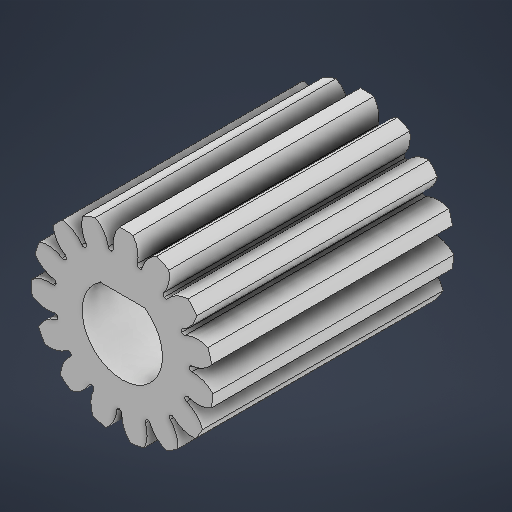
# Autodesk Inventor part: piñon
Saved by Autodesk Inventor 2025.3 (Build 293356000, 356)
## iProperties
Created: 2024-05-16
Part Number: piñon
Material: Genérico
Document SubType Name: Modeling
Designer: Jonathan Galarza
Density: 1 g/cm^3
Appearance: Valor por defecto
Author: Jonathan Galarza
Title: Eje piñon
Autodesk Inventor part; units mm, degrees
ref_plane "YZ Plane" through (0, 0, 0) normal (1, 0, 0) x (0, 1, 0)
ref_plane "XZ Plane" through (0, 0, 0) normal (0, 1, 0) x (-1, 0, 0)
ref_plane "XY Plane" through (0, 0, 0) normal (0, 0, 1) x (1, 0, 0)
sketch "Boceto1" plane through (0, 0, 0) normal (0, 0, 1) x (1, 0, 0)
  circle A0 centre (0, 0) radius 17
  dimension "d0" = 34
  constraints: 1 centre point, 1 coincident
  measures "d0" diameter of A0
extrude "Extrusión1" add sketch "Boceto1" along normal blind 1
sketch "Boceto2" plane through (0, 0, 0) normal (0, 0, -1) x (-1, 0, 0)
  point P0 (0, 0)
sketch "Boceto6" plane through (0, 0, 1) normal (0, 0, 1) x (1, 0, 0)
  arc A0 (6.6315, -1.5044) -> (6.7809, -0.5097) centre (0, 0) ccw
  circle A1 centre (0, 0) radius 5
  line L0 (0, 0) -> (6.8, 0) construction
  line L1 (0, 0) -> (6.1907, 0) construction
  arc A2 (6.7809, -0.5097) -> (4.999, 0.1018) centre (5.2981, -1.9284) ccw
  line L2 (0, 0) -> (6.2602, 0) construction
  arc A3 (4.7486, -1.5656) -> (6.6315, -1.5044) centre (5.6308, 0.2872) ccw
  arc A4 (6.4019, 2.2924) -> (4.5254, 2.1263) centre (5.6244, 0.3933) ccw
  arc A5 (6.6701, 1.3229) -> (6.4019, 2.2924) centre (0, 0) ccw
  arc A6 (4.9748, 0.5012) -> (6.6701, 1.3229) centre (5.0272, 2.5527) ccw
  arc A7 (4.916, 4.6981) -> (3.2693, 3.7831) centre (4.9782, 2.647) ccw
  arc A8 (5.5553, 3.9215) -> (4.916, 4.6981) centre (0, 0) ccw
  arc A9 (4.3409, 2.4813) -> (5.5553, 3.9215) centre (3.5543, 4.3767) ccw
  arc A10 (2.5801, 6.2915) -> (1.4479, 4.7858) centre (3.4712, 4.4429) ccw
  arc A11 (3.48, 5.842) -> (2.5801, 6.2915) centre (0, 0) ccw
  arc A12 (2.9563, 4.0324) -> (3.48, 5.842) centre (1.4669, 5.444) ccw
  arc A13 (-0.2019, 6.797) -> (-0.6238, 4.9609) centre (1.364, 5.4707) ccw
  arc A14 (0.803, 6.7524) -> (-0.2019, 6.797) centre (0, 0) ccw
  arc A15 (1.0606, 4.8862) -> (0.803, 6.7524) centre (-0.8742, 5.57) ccw
  arc A16 (-2.949, 6.1272) -> (-2.5877, 4.2783) centre (-0.9791, 5.5525) ccw
  arc A17 (-2.0129, 6.4952) -> (-2.949, 6.1272) centre (0, 0) ccw
  arc A18 (-1.0185, 4.8952) -> (-2.0129, 6.4952) centre (-3.0642, 4.7328) ccw
  arc A19 (-5.1863, 4.398) -> (-4.1041, 2.8559) centre (-3.1528, 4.6742) ccw
  arc A20 (-4.4807, 5.115) -> (-5.1863, 4.398) centre (0, 0) ccw
  arc A21 (-2.9215, 4.0577) -> (-4.4807, 5.115) centre (-4.7243, 3.0774) ccw
  arc A22 (-6.5267, 1.9084) -> (-4.9109, 0.9397) centre (-4.7814, 2.9878) ccw
  arc A23 (-6.1738, 2.8503) -> (-6.5267, 1.9084) centre (0, 0) ccw
  arc A24 (-4.3193, 2.5186) -> (-6.1738, 2.8503) centre (-5.5675, 0.8898) ccw
  arc A25 (-6.7387, -0.9113) -> (-4.8686, -1.139) centre (-5.5833, 0.7847) ccw
  arc A26 (-6.7994, 0.0928) -> (-6.7387, -0.9113) centre (0, 0) ccw
  arc A27 (-4.9703, 0.5441) -> (-6.7994, 0.0928) centre (-5.4481, -1.4517) ccw
  arc A28 (-5.7854, -3.5734) -> (-3.9844, -3.0207) centre (-5.4197, -1.5541) ccw
  arc A29 (-6.2493, -2.6808) -> (-5.7854, -3.5734) centre (0, 0) ccw
  arc A30 (-4.7619, -1.5246) -> (-6.2493, -2.6808) centre (-4.3866, -3.5421) ccw
  arc A31 (-3.8318, -5.6176) -> (-2.4113, -4.3801) centre (-4.3191, -3.6241) ccw
  arc A32 (-4.6186, -4.9909) -> (-3.8318, -5.6176) centre (0, 0) ccw
  arc A33 (-3.7301, -3.3296) -> (-4.6186, -4.9909) centre (-2.5667, -5.0201) ccw
  arc A34 (-1.2157, -6.6905) -> (-0.4213, -4.9822) centre (-2.4716, -5.0675) ccw
  arc A35 (-2.1893, -6.4379) -> (-1.2157, -6.6905) centre (0, 0) ccw
  arc A36 (-2.0534, -4.5589) -> (-2.1893, -6.4379) centre (-0.3029, -5.63) ccw
  arc A37 (1.6107, -6.6065) -> (1.6416, -4.7228) centre (-0.1968, -5.6347) ccw
  arc A38 (0.6185, -6.7718) -> (1.6107, -6.6065) centre (0, 0) ccw
  arc A39 (-0.0216, -5) -> (0.6185, -6.7718) centre (2.0132, -5.2665) ccw
  arc A40 (4.1585, -5.3802) -> (3.4206, -3.6468) centre (2.1121, -5.2276) ccw
  arc A41 (3.3194, -5.9348) -> (4.1585, -5.3802) centre (0, 0) ccw
  arc A42 (2.014, -4.5765) -> (3.3194, -5.9348) centre (3.9812, -3.9923) ccw
  arc A43 (5.9873, -3.2236) -> (4.6082, -1.9402) centre (4.0557, -3.9166) ccw
  arc A44 (5.4463, -4.0716) -> (5.9873, -3.2236) centre (0, 0) ccw
  arc A45 (3.7013, -3.3616) -> (5.4463, -4.0716) centre (5.2608, -2.0279) ccw
  point P0 (-4.1041, 2.8559)
  point P1 (-4.9109, 0.9397)
  point P2 (-4.9703, 0.5441)
  point P3 (-4.8686, -1.139)
  point P4 (-4.7619, -1.5246)
  point P5 (-3.9844, -3.0207)
  point P6 (-0.4213, -4.9822)
  point P7 (1.6416, -4.7228)
  point P8 (3.4206, -3.6468)
  point P9 (4.6082, -1.9402)
  point P10 (4.5254, 2.1263)
  point P11 (3.2693, 3.7831)
  point P12 (2.9563, 4.0324)
  point P13 (1.4479, 4.7858)
  point P14 (1.0606, 4.8862)
  point P15 (-0.6238, 4.9609)
  dimension "d46" = 10
  dimension "d17" = 360
  constraints: 90 point on circle, 45 centre point, 6 end point, 3 coincident, 3 horizontal, 152 other
extrude "Extrusión4" add sketch "Boceto6" along normal blind 19
fillet "Empalme2" radius 0.2 2 edges at (1.0606, 4.8862, 10.5) (1.4479, 4.7858, 10.5)
pattern_circular "Patrón circular2" count 15 over 360 about axis through (0, 0, 0) along (0, 0, 1) of "Empalme2"
sketch "Boceto8" plane through (0, 0, 0) normal (0, 0, -1) x (-1, 0, 0)
  circle A0 centre (0, 0) radius 17 projected
  circle A1 centre (0, 0) radius 17 projected
  circle A2 centre (0, 0) radius 17 projected
  arc A3 (2.7047, 4.4419) -> (2.949, 6.1272) centre (0.9791, 5.5525) ccw projected
  arc A4 (2.7047, 4.4419) -> (2.7509, 4.1752) centre (2.8729, 4.3337) ccw projected
  arc A5 (2.7509, 4.1752) -> (3.0264, 4.2299) centre (2.8609, 4.3423) ccw projected
  arc A6 (4.4807, 5.115) -> (3.0264, 4.2299) centre (4.7243, 3.0774) ccw projected
  arc A7 (5.1863, 4.398) -> (4.4807, 5.115) centre (0, 0) ccw projected
  arc A8 (4.2776, 2.9578) -> (5.1863, 4.398) centre (3.1528, 4.6742) ccw projected
  arc A9 (4.2776, 2.9578) -> (4.2113, 2.6954) centre (4.3872, 2.7905) ccw projected
  arc A10 (4.2113, 2.6954) -> (4.4852, 2.6333) centre (4.3797, 2.8032) ccw projected
  arc A11 (6.1738, 2.8503) -> (4.4852, 2.6333) centre (5.5675, 0.8898) ccw projected
  arc A12 (6.5267, 1.9084) -> (6.1738, 2.8503) centre (0, 0) ccw projected
  arc A13 (5.1108, 0.9623) -> (6.5267, 1.9084) centre (4.7814, 2.9878) ccw projected
  arc A14 (5.1108, 0.9623) -> (4.9435, 0.7495) centre (5.1429, 0.7648) ccw projected
  arc A15 (4.9435, 0.7495) -> (5.1685, 0.5813) centre (5.1412, 0.7795) ccw projected
  arc A16 (6.7994, 0.0928) -> (5.1685, 0.5813) centre (5.4481, -1.4517) ccw projected
  arc A17 (6.7387, -0.9113) -> (6.7994, 0.0928) centre (0, 0) ccw projected
  arc A18 (5.0603, -1.1997) -> (6.7387, -0.9113) centre (5.5833, 0.7847) ccw projected
  arc A19 (5.0603, -1.1997) -> (4.821, -1.326) centre (5.0094, -1.3931) ccw projected
  arc A20 (4.821, -1.326) -> (4.9581, -1.5711) centre (5.0138, -1.3791) ccw projected
  arc A21 (6.2493, -2.6808) -> (4.9581, -1.5711) centre (4.3866, -3.5421) ccw projected
  arc A22 (5.7854, -3.5734) -> (6.2493, -2.6808) centre (0, 0) ccw projected
  arc A23 (4.1349, -3.1542) -> (5.7854, -3.5734) centre (5.4197, -1.5541) ccw projected
  arc A24 (4.1349, -3.1542) -> (3.8648, -3.1722) centre (4.0097, -3.3101) ccw projected
  arc A25 (3.8648, -3.1722) -> (3.8904, -3.452) centre (4.0194, -3.2991) ccw projected
  arc A26 (4.6186, -4.9909) -> (3.8904, -3.452) centre (2.5667, -5.0201) ccw projected
  arc A27 (3.8318, -5.6176) -> (4.6186, -4.9909) centre (0, 0) ccw projected
  arc A28 (2.4945, -4.5633) -> (3.8318, -5.6176) centre (4.3191, -3.6241) ccw projected
  arc A29 (2.4945, -4.5633) -> (2.2404, -4.47) centre (2.3167, -4.6549) ccw projected
  arc A30 (2.2404, -4.47) -> (2.15, -4.7359) centre (2.33, -4.6487) ccw projected
  arc A31 (2.1893, -6.4379) -> (2.15, -4.7359) centre (0.3029, -5.63) ccw projected
  arc A32 (1.2157, -6.6905) -> (2.1893, -6.4379) centre (0, 0) ccw projected
  arc A33 (0.4228, -5.1834) -> (1.2157, -6.6905) centre (2.4716, -5.0675) ccw projected
  arc A34 (0.4228, -5.1834) -> (0.2286, -4.9948) centre (0.2231, -5.1947) ccw projected
  arc A35 (0.2286, -4.9948) -> (0.0379, -5.2009) centre (0.2378, -5.1946) ccw projected
  arc A36 (-0.6185, -6.7718) -> (0.0379, -5.2009) centre (-2.0132, -5.2665) ccw projected
  arc A37 (-1.6107, -6.6065) -> (-0.6185, -6.7718) centre (0, 0) ccw projected
  arc A38 (-1.7221, -4.9072) -> (-1.6107, -6.6065) centre (0.1968, -5.6347) ccw projected
  arc A39 (-1.7221, -4.9072) -> (-1.8227, -4.6559) centre (-1.9091, -4.8363) ccw projected
  arc A40 (-1.8227, -4.6559) -> (-2.0808, -4.7667) centre (-1.8956, -4.8422) ccw projected
  arc A41 (-3.3194, -5.9348) -> (-2.0808, -4.7667) centre (-3.9812, -3.9923) ccw projected
  arc A42 (-4.1585, -5.3802) -> (-3.3194, -5.9348) centre (0, 0) ccw projected
  arc A43 (-3.5691, -3.7825) -> (-4.1585, -5.3802) centre (-2.1121, -5.2276) ccw projected
  arc A44 (-3.5691, -3.7825) -> (-3.5588, -3.5121) centre (-3.7111, -3.6417) ccw projected
  arc A45 (-3.5588, -3.5121) -> (-3.8397, -3.5083) centre (-3.7012, -3.6526) ccw projected
  arc A46 (-5.4463, -4.0716) -> (-3.8397, -3.5083) centre (-5.2608, -2.0279) ccw projected
  arc A47 (-5.9873, -3.2236) -> (-5.4463, -4.0716) centre (0, 0) ccw projected
  arc A48 (-4.7991, -2.0038) -> (-5.9873, -3.2236) centre (-4.0557, -3.9166) ccw projected
  arc A49 (-4.7991, -2.0038) -> (-4.6797, -1.7609) centre (-4.8715, -1.8174) ccw projected
  arc A50 (-4.6797, -1.7609) -> (-4.9347, -1.6432) centre (-4.8668, -1.8314) ccw projected
  arc A51 (-6.6315, -1.5044) -> (-4.9347, -1.6432) centre (-5.6308, 0.2872) ccw projected
  arc A52 (-6.7809, -0.5097) -> (-6.6315, -1.5044) centre (0, 0) ccw projected
  arc A53 (-5.1992, 0.1214) -> (-6.7809, -0.5097) centre (-5.2981, -1.9284) ccw projected
  arc A54 (-5.1992, 0.1214) -> (-4.9913, 0.2947) centre (-5.1896, 0.3211) ccw projected
  arc A55 (-4.9913, 0.2947) -> (-5.1764, 0.506) centre (-5.191, 0.3065) ccw projected
  arc A56 (-6.6701, 1.3229) -> (-5.1764, 0.506) centre (-5.0272, 2.5527) ccw projected
  arc A57 (-6.4019, 2.2924) -> (-6.6701, 1.3229) centre (0, 0) ccw projected
  arc A58 (-4.7003, 2.2256) -> (-6.4019, 2.2924) centre (-5.6244, 0.3933) ccw projected
  arc A59 (-4.7003, 2.2256) -> (-4.4399, 2.2994) centre (-4.6103, 2.4042) ccw projected
  arc A60 (-4.4399, 2.2994) -> (-4.5231, 2.5677) centre (-4.6175, 2.3913) ccw projected
  arc A61 (-5.5553, 3.9215) -> (-4.5231, 2.5677) centre (-3.5543, 4.3767) ccw projected
  arc A62 (-4.916, 4.6981) -> (-5.5553, 3.9215) centre (0, 0) ccw projected
  arc A63 (-3.3887, 3.945) -> (-4.916, 4.6981) centre (-4.9782, 2.647) ccw projected
  arc A64 (-3.3887, 3.945) -> (-3.1208, 3.9065) centre (-3.2338, 4.0715) ccw projected
  arc A65 (-3.1208, 3.9065) -> (-3.0877, 4.1854) centre (-3.2457, 4.0627) ccw projected
  arc A66 (-3.48, 5.842) -> (-3.0877, 4.1854) centre (-1.4669, 5.444) ccw projected
  arc A67 (-2.5801, 6.2915) -> (-3.48, 5.842) centre (0, 0) ccw projected
  arc A68 (-1.4912, 4.9822) -> (-2.5801, 6.2915) centre (-3.4712, 4.4429) ccw projected
  arc A69 (-1.4912, 4.9822) -> (-1.2621, 4.8381) centre (-1.2982, 5.0348) ccw projected
  arc A70 (-1.2621, 4.8381) -> (-1.1184, 5.0794) centre (-1.3126, 5.0316) ccw projected
  arc A71 (-0.803, 6.7524) -> (-1.1184, 5.0794) centre (0.8742, 5.57) ccw projected
  arc A72 (0.2019, 6.797) -> (-0.803, 6.7524) centre (0, 0) ccw projected
  arc A73 (0.6642, 5.158) -> (0.2019, 6.797) centre (-1.364, 5.4707) ccw projected
  arc A74 (0.6642, 5.158) -> (0.8148, 4.9332) centre (0.8618, 5.1276) ccw projected
  arc A75 (0.8148, 4.9332) -> (1.0443, 5.0952) centre (0.8474, 5.1305) ccw projected
  arc A76 (2.0129, 6.4952) -> (1.0443, 5.0952) centre (3.0642, 4.7328) ccw projected
  arc A77 (2.949, 6.1272) -> (2.0129, 6.4952) centre (0, 0) ccw projected
  point P0 (5.0323, 16.2381)
  point P1 (0.5048, 16.9925)
  point P2 (11.2018, 12.7874)
  point P3 (7.3726, 15.3181)
  point P4 (15.4345, 7.1257)
  point P5 (12.9657, 10.9951)
  point P6 (16.9984, 0.2319)
  point P7 (16.3168, 4.7709)
  point P8 (15.6231, -6.702)
  point P9 (16.8467, -2.2782)
  point P10 (11.5465, -12.4771)
  point P11 (14.4635, -8.9334)
  point P12 (5.4733, -16.0948)
  point P13 (9.5796, -14.0439)
  point P14 (-1.5462, -16.9295)
  point P15 (3.0392, -16.7261)
  point P16 (-8.2984, -14.837)
  point P17 (-4.0267, -16.5162)
  point P18 (-13.6157, -10.179)
  point P19 (-10.3963, -13.4505)
  point P20 (-16.5788, -3.761)
  point P21 (-14.9683, -8.0591)
  point P22 (-16.6752, 3.3074)
  point P23 (-16.9522, -1.2742)
  point P24 (-13.8883, 9.8038)
  point P25 (-16.0048, 5.7311)
  point P26 (-8.7, 14.6051)
  point P27 (-12.2901, 11.7453)
  point P28 (-2.0074, 16.8811)
  point P29 (-6.4503, 15.7287)
  constraints: 1 other
extrude "Extrusión6" cut sketch "Boceto8" against normal blind 2 contours A0 | A4 A5 A6 A7 A8 A9 A10 A11 A12 A13 A14 A15 A16 A17 A18 A19 A20 A21 A22 A23 A24 A25 A26 A27 A28 A29 A30 A31 A32 A33 A34 A35 A36 A37 A38 A39 A40 A41 A42 A43 A44 A45 A46 A47 A48 A49 A50 A51 A52 A53 A54 A55 A56 A57 A58 A59 A60 A61 A62 A63 A64 A65 A66 A67 A68 A69 A70 A71 A72 A73 A74 A75 A76 A77 A3
sketch "Boceto9" plane through (0, 0, 20) normal (0, 0, 1) x (1, 0, 0)
  circle A0 centre (0, 0) radius 3
  line L0 (0, 0) -> (0, 2.5) construction
  line L1 (0, 2.5) -> (-1.6583, 2.5)
  line L2 (0, 2.5) -> (1.6583, 2.5)
  dimension "d42" = 6
  dimension "d43" = 2.5
  constraints: 6 end point, 2 point on circle, 1 centre point, 1 coincident, 1 horizontal, 1 point on line, 1 vertical
  measures "d42" diameter of A0
  measures "d43" distance of L0.start L0.end
extrude "Extrusión7" cut sketch "Boceto9" against normal through all contours A0 L1 L2 picked at (-0.014, -1.1519)
